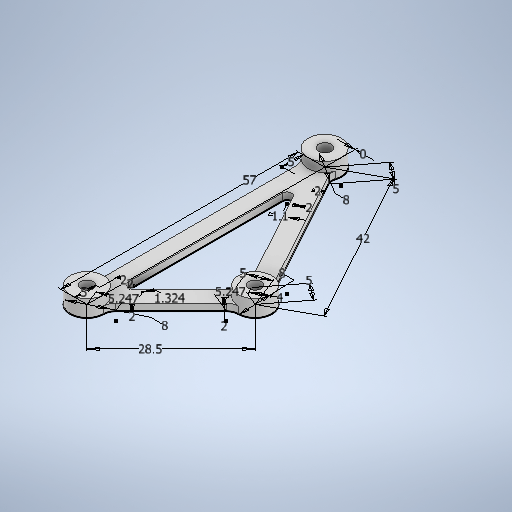
# Autodesk Inventor part: A2P2
Saved by Autodesk Inventor 2025.2 (Build 292293000, 293)
## iProperties
Created: 2025-05-22
Part Number: A2P2
Material: Generic
Document SubType Name: Sheet Metal
Designer: Admin
Density: 1 g/cm^3
Sheet Metal Rule: Default
Appearance: Default
Author: Admin
Autodesk Inventor part; units mm, degrees
ref_plane "YZ Plane" through (0, 0, 0) normal (1, 0, 0) x (0, 1, 0)
ref_plane "XZ Plane" through (0, 0, 0) normal (0, 1, 0) x (-1, 0, 0)
ref_plane "XY Plane" through (0, 0, 0) normal (0, 0, 1) x (1, 0, 0)
sketch "Sketch1" plane through (0, 0, 0) normal (0, 1, 0) x (-1, 0, 0)
  circle A0 centre (0, 0) radius 4
  line L0 (2, -5) -> (2, -52)
  line L1 (-2, -8.025) -> (-2, -44.8708)
  circle A1 centre (0, -57) radius 4
  circle A2 centre (-20.1538, -20.1513) radius 4
  line L2 (-4.2607, -7.0885) -> (-15.4991, -18.3254)
  line L3 (-4.8445, -2.0156) -> (-18.1376, -15.3071)
  line L4 (-16.2001, -23.2121) -> (-4.0655, -45.3988)
  line L5 (-19.7095, -25.1315) -> (-3.9537, -53.9392)
  arc A3 (2.8966, -2.7586) -> (2, -5) centre (5.25, -5) ccw
  arc A4 (2, -52) -> (2.8966, -54.2414) centre (5.25, -52) ccw
  arc A5 (-4.8445, -2.0156) -> (-4, 0.0134) centre (-6.8829, 0.023) ccw
  arc A6 (-20.1666, -16.1513) -> (-18.1376, -15.3071) centre (-20.1759, -13.2686) ccw
  line L6 (0, 0) -> (-20.1538, -20.1513) construction
  line L7 (-20.1538, -20.1513) -> (0, -57) construction
  arc A7 (-15.4991, -18.3254) -> (-16.1566, -20.0011) centre (-13.9082, -19.9165) ccw
  arc A8 (-16.36, -21.4193) -> (-16.2001, -23.2121) centre (-14.2261, -22.1325) ccw
  arc A9 (-2, -8.025) -> (-4.2607, -7.0885) centre (-3.3243, -8.025) ccw
  arc A10 (-4.0655, -45.3988) -> (-2, -44.8708) centre (-3.1002, -44.8708) ccw
  arc A11 (-19.7095, -25.1315) -> (-21.1328, -24.0296) centre (-21.6835, -26.2112) ccw
  arc A12 (-3.7937, -55.7321) -> (-3.9537, -53.9392) centre (-5.9277, -55.0188) ccw
  dimension "d0" = 8
  dimension "d1" = 8
  dimension "d2" = 8
  dimension "d3" = 57
  dimension "d4" = 42
  dimension "d5" = 28.5
  dimension "d6" = 2
  dimension "d7" = 2
  dimension "d8" = 5
  dimension "d10" = 5
  dimension "d11" = 0
  dimension "d12" = 5.2471
  dimension "d14" = 5.247
  dimension "d15" = 2
  dimension "d16" = 2
  dimension "d17" = 2
  dimension "d18" = 2
  dimension "d19" = 4
  dimension "d20" = 5
  dimension "d21" = 5
  dimension "d22" = 5
  dimension "d23" = 1.1002
  dimension "d24" = 1.3243
  constraints: 28 point on circle, 20 tangent, 16 end point, 13 centre point, 4 parallel, 2 vertical, 1 coincident
  measures "d0" diameter of A0
  measures "d1" diameter of A1
  measures "d2" diameter of A2
  measures "d3" distance of L7.end point (0, 0)
  measures "d4" distance of L6.end L7.end
  measures "d5" distance of point (0, 0) L6.end
  measures "d6" horizontal distance of point (0, 0) L0.start
  measures "d7" horizontal distance of point (0, 0) L1.start
  measures "d8" vertical distance of point (0, 0) L0.start
  measures "d10" vertical distance of L7.end L0.end
  measures "d11" horizontal distance of L7.end point (0, 0)
  measures "d12" distance of L3.start point (0, 0)
  measures "d14" distance of L6.end L3.end
  measures "d15" distance from line of L6 L3.start
  measures "d16" distance from line of L6 L2.end
  measures "d17" distance from line of L7 L4.end
  measures "d18" distance from line of L7 L5.end
  measures "d19" distance of L4.start L5.start
  measures "d20" distance of L5.end L7.end
  measures "d21" distance of L6.end L4.start
  measures "d22" distance of L6.end L2.end
  measures "d23" distance from line of L4 A10.centre
  measures "d24" radius of A9
extrude "Extrusion1" add sketch "Sketch1" along normal blind 4 contours A0 | A2 | A1
extrude "Extrusion2" add sketch "Sketch1" along normal blind 1.7 contours A0 A3 L0 A4 A1 A12 L5 A11 A2 A8 L4 A10 L1 A9 L2 A7 A6 L3 A5
sketch "Sketch2" plane through (0, 4, 0) normal (0, 1, 0) x (1, 0, 0)
  circle A0 centre (0, 0) radius 4 projected
  circle A1 centre (0, 0) radius 1.5
  circle A2 centre (20.1538, 20.1513) radius 4 projected
  circle A3 centre (20.1538, 20.1513) radius 1.5
  circle A4 centre (0, 57.0468) radius 1.5
  dimension "d29" = 3
  dimension "d30" = 3
  dimension "d31" = 3
  constraints: 3 centre point, 2 coincident
  measures "d29" diameter of A1
  measures "d30" diameter of A4
  measures "d31" diameter of A3
extrude "Extrusion3" cut sketch "Sketch2" against normal blind 4 contours A1 | A3 | A4
equation "\"BendRadius\" = Thickness"
equation "\"BendReliefWidth\" = Thickness"
equation "\"BendReliefDepth\" = 0.5 * Thickness"
equation "\"CornerReliefSize\" = 4 * Thickness"
equation "\"MinimumRemnant\" = 2 * Thickness"
equation "\"TransitionRadius\" = BendRadius"
equation "\"JacobiRadiusSize\" = BendRadius"
equation "\"GapSize\" = Thickness"
equation "\"Thickness\" = 3.048"
body "Solid1"
